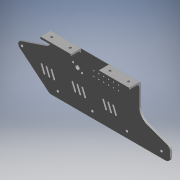
# Autodesk Inventor part: platform_track_support
Saved by Autodesk Inventor 2019 (Build 230136000, 136)
## iProperties
Part Number: platform_track_support
Material: Generic
Document SubType Name: Modeling
Designer: Jorge
Appearance: Default
Author: Jorge
Autodesk Inventor part; units mm, degrees
ref_plane "YZ Plane" through (0, 0, 0) normal (1, 0, 0) x (0, 1, 0)
ref_plane "XZ Plane" through (0, 0, 0) normal (0, 1, 0) x (-1, 0, 0)
ref_plane "XY Plane" through (0, 0, 0) normal (0, 0, 1) x (1, 0, 0)
sketch "Sketch1" plane through (0, 0, 0) normal (0, 0, 1) x (1, 0, 0)
  line L0 (2.505, 0) -> (188, 0)
  line L1 (195, 7) -> (195, 17.0802)
  line L2 (190.371, 23.6664) -> (158.2256, 35.2388)
  line L3 (145, 54.0565) -> (145, 89)
  line L4 (145, 89) -> (1.5, 89)
  line L5 (1.5, 89) -> (1.5, 73.7111)
  line L6 (-5.3421, 64.2228) -> (-46.8948, 50.393)
  line L7 (-1.9362, 1.5893) -> (-48.8068, 40.0623)
  arc A0 (-46.8948, 50.393) -> (-48.8068, 40.0623) centre (-45, 44.7) ccw
  arc A1 (-1.9362, 1.5893) -> (2.505, 0) centre (2.505, 7) ccw
  arc A2 (188, 0) -> (195, 7) centre (188, 7) ccw
  arc A3 (195, 17.0802) -> (190.371, 23.6664) centre (188, 17.0802) ccw
  arc A4 (145, 54.0565) -> (158.2256, 35.2388) centre (165, 54.0565) ccw
  arc A5 (-5.3421, 64.2228) -> (1.5, 73.7111) centre (-8.5, 73.7111) ccw
  line L8 (13, 10) -> (181, 10) construction
  circle A6 centre (13, 10) radius 2
  circle A7 centre (181, 10) radius 2
  circle A8 centre (69, 10) radius 2
  circle A9 centre (125, 10) radius 2
  circle A10 centre (-45, 44.7) radius 2
  circle A11 centre (45, 59.2) radius 3.5
  circle A12 centre (52.2081, 55.1868) radius 1.75
  line L9 (52.2081, 55.1868) -> (48.058, 57.4974) construction
  circle A13 centre (37.7919, 63.2132) radius 1.75
  line L10 (41.942, 60.9026) -> (37.7919, 63.2132) construction
  line L11 (48.058, 57.4974) -> (41.942, 60.9026) construction
  arc A14 (-11.7614, 35.5207) -> (-14.5469, 34.4068) centre (-13.1542, 34.9637) ccw
  arc A15 (-9.2558, 25.2142) -> (-10.0917, 23.2645) centre (-8.6989, 23.8214) ccw construction
  line L12 (-13.1542, 34.9637) -> (-8.6989, 23.8214) construction
  line L13 (-14.5469, 34.4068) -> (-10.0917, 23.2645)
  line L14 (-7.3061, 24.3784) -> (-11.7614, 35.5207)
  arc A16 (-7.3061, 24.3784) -> (-9.2558, 25.2142) centre (-8.6989, 23.8214) ccw construction
  arc A17 (-10.0917, 23.2645) -> (-7.3061, 24.3784) centre (-8.6989, 23.8214) ccw
  arc A18 (-12.5973, 33.571) -> (-11.7614, 35.5207) centre (-13.1542, 34.9637) ccw construction
  arc A19 (-14.5469, 34.4068) -> (-12.5973, 33.571) centre (-13.1542, 34.9637) ccw construction
  line L15 (-10.9265, 29.3926) -> (151.0905, 29.3926) construction
  arc A20 (-4.5973, 33.571) -> (-3.7614, 35.5207) centre (-5.1542, 34.9637) ccw construction
  arc A21 (-6.5469, 34.4068) -> (-4.5973, 33.571) centre (-5.1542, 34.9637) ccw construction
  arc A22 (-3.7614, 35.5207) -> (-6.5469, 34.4068) centre (-5.1542, 34.9637) ccw
  arc A23 (0.6939, 24.3784) -> (-1.2558, 25.2142) centre (-0.6989, 23.8214) ccw construction
  arc A24 (-2.0917, 23.2645) -> (0.6939, 24.3784) centre (-0.6989, 23.8214) ccw
  arc A25 (-1.2558, 25.2142) -> (-2.0917, 23.2645) centre (-0.6989, 23.8214) ccw construction
  line L16 (0.6939, 24.3784) -> (-3.7614, 35.5207)
  line L17 (-6.5469, 34.4068) -> (-2.0917, 23.2645)
  arc A26 (3.4027, 33.571) -> (4.2386, 35.5207) centre (2.8458, 34.9637) ccw construction
  arc A27 (1.4531, 34.4068) -> (3.4027, 33.571) centre (2.8458, 34.9637) ccw construction
  arc A28 (4.2386, 35.5207) -> (1.4531, 34.4068) centre (2.8458, 34.9637) ccw
  arc A29 (8.6939, 24.3784) -> (6.7442, 25.2142) centre (7.3011, 23.8214) ccw construction
  arc A30 (5.9083, 23.2645) -> (8.6939, 24.3784) centre (7.3011, 23.8214) ccw
  arc A31 (6.7442, 25.2142) -> (5.9083, 23.2645) centre (7.3011, 23.8214) ccw construction
  line L18 (8.6939, 24.3784) -> (4.2386, 35.5207)
  line L19 (1.4531, 34.4068) -> (5.9083, 23.2645)
  arc A32 (54.2386, 35.5207) -> (51.4531, 34.4068) centre (52.8458, 34.9637) ccw
  arc A33 (53.4027, 33.571) -> (54.2386, 35.5207) centre (52.8458, 34.9637) ccw construction
  arc A34 (46.2386, 35.5207) -> (43.4531, 34.4068) centre (44.8458, 34.9637) ccw
  arc A35 (51.4531, 34.4068) -> (53.4027, 33.571) centre (52.8458, 34.9637) ccw construction
  line L20 (58.6939, 24.3784) -> (54.2386, 35.5207)
  line L21 (51.4531, 34.4068) -> (55.9083, 23.2645)
  line L22 (50.6939, 24.3784) -> (46.2386, 35.5207)
  line L23 (43.4531, 34.4068) -> (47.9083, 23.2645)
  arc A36 (45.4027, 33.571) -> (46.2386, 35.5207) centre (44.8458, 34.9637) ccw construction
  arc A37 (43.4531, 34.4068) -> (45.4027, 33.571) centre (44.8458, 34.9637) ccw construction
  arc A38 (38.2386, 35.5207) -> (35.4531, 34.4068) centre (36.8458, 34.9637) ccw
  line L24 (36.8458, 34.9637) -> (41.3011, 23.8214) construction
  line L25 (35.4531, 34.4068) -> (39.9083, 23.2645)
  line L26 (42.6939, 24.3784) -> (38.2386, 35.5207)
  arc A39 (37.4027, 33.571) -> (38.2386, 35.5207) centre (36.8458, 34.9637) ccw construction
  arc A40 (35.4531, 34.4068) -> (37.4027, 33.571) centre (36.8458, 34.9637) ccw construction
  arc A41 (58.6939, 24.3784) -> (56.7442, 25.2142) centre (57.3011, 23.8214) ccw construction
  arc A42 (55.9083, 23.2645) -> (58.6939, 24.3784) centre (57.3011, 23.8214) ccw
  arc A43 (56.7442, 25.2142) -> (55.9083, 23.2645) centre (57.3011, 23.8214) ccw construction
  arc A44 (48.7442, 25.2142) -> (47.9083, 23.2645) centre (49.3011, 23.8214) ccw construction
  arc A45 (42.6939, 24.3784) -> (40.7442, 25.2142) centre (41.3011, 23.8214) ccw construction
  arc A46 (40.7442, 25.2142) -> (39.9083, 23.2645) centre (41.3011, 23.8214) ccw construction
  arc A47 (50.6939, 24.3784) -> (48.7442, 25.2142) centre (49.3011, 23.8214) ccw construction
  arc A48 (47.9083, 23.2645) -> (50.6939, 24.3784) centre (49.3011, 23.8214) ccw
  arc A49 (39.9083, 23.2645) -> (42.6939, 24.3784) centre (41.3011, 23.8214) ccw
  arc A50 (104.2386, 35.5207) -> (101.4531, 34.4068) centre (102.8458, 34.9637) ccw
  arc A51 (103.4027, 33.571) -> (104.2386, 35.5207) centre (102.8458, 34.9637) ccw construction
  arc A52 (96.2386, 35.5207) -> (93.4531, 34.4068) centre (94.8458, 34.9637) ccw
  arc A53 (101.4531, 34.4068) -> (103.4027, 33.571) centre (102.8458, 34.9637) ccw construction
  line L27 (108.6939, 24.3784) -> (104.2386, 35.5207)
  line L28 (101.4531, 34.4068) -> (105.9083, 23.2645)
  line L29 (100.6939, 24.3784) -> (96.2386, 35.5207)
  line L30 (93.4531, 34.4068) -> (97.9083, 23.2645)
  arc A54 (95.4027, 33.571) -> (96.2386, 35.5207) centre (94.8458, 34.9637) ccw construction
  arc A55 (93.4531, 34.4068) -> (95.4027, 33.571) centre (94.8458, 34.9637) ccw construction
  arc A56 (88.2386, 35.5207) -> (85.4531, 34.4068) centre (86.8458, 34.9637) ccw
  line L31 (86.8458, 34.9637) -> (91.3011, 23.8214) construction
  line L32 (85.4531, 34.4068) -> (89.9083, 23.2645)
  line L33 (92.6939, 24.3784) -> (88.2386, 35.5207)
  arc A57 (87.4027, 33.571) -> (88.2386, 35.5207) centre (86.8458, 34.9637) ccw construction
  arc A58 (85.4531, 34.4068) -> (87.4027, 33.571) centre (86.8458, 34.9637) ccw construction
  arc A59 (108.6939, 24.3784) -> (106.7442, 25.2142) centre (107.3011, 23.8214) ccw construction
  arc A60 (105.9083, 23.2645) -> (108.6939, 24.3784) centre (107.3011, 23.8214) ccw
  arc A61 (106.7442, 25.2142) -> (105.9083, 23.2645) centre (107.3011, 23.8214) ccw construction
  arc A62 (98.7442, 25.2142) -> (97.9083, 23.2645) centre (99.3011, 23.8214) ccw construction
  arc A63 (92.6939, 24.3784) -> (90.7442, 25.2142) centre (91.3011, 23.8214) ccw construction
  arc A64 (90.7442, 25.2142) -> (89.9083, 23.2645) centre (91.3011, 23.8214) ccw construction
  arc A65 (100.6939, 24.3784) -> (98.7442, 25.2142) centre (99.3011, 23.8214) ccw construction
  arc A66 (97.9083, 23.2645) -> (100.6939, 24.3784) centre (99.3011, 23.8214) ccw
  arc A67 (89.9083, 23.2645) -> (92.6939, 24.3784) centre (91.3011, 23.8214) ccw
  circle A68 centre (111.4036, 67.8621) radius 1
  line L34 (111.4036, 67.8621) -> (111.4036, 49.7064) construction
  line L35 (111.4036, 67.8621) -> (82.8465, 67.8621) construction
  circle A69 centre (111.4036, 59.8621) radius 1
  circle A70 centre (103.4036, 67.8621) radius 1
  circle A71 centre (103.4036, 59.8621) radius 1
  circle A72 centre (95.4036, 67.8621) radius 1
  circle A73 centre (95.4036, 59.8621) radius 1
  circle A74 centre (87.4036, 67.8621) radius 1
  circle A75 centre (87.4036, 59.8621) radius 1
  circle A76 centre (79.4036, 67.8621) radius 1
  circle A77 centre (79.4036, 59.8621) radius 1
  circle A78 centre (71.4036, 67.8621) radius 1
  circle A79 centre (71.4036, 59.8621) radius 1
  circle A80 centre (45, 59.2) radius 12.5 construction
  point P0 (0, 0)
  point P1 (0, 0)
  point P2 (195, 0)
  point P3 (195, 22)
  point P4 (145, 40)
  point P5 (1.5, 66.5)
  point P6 (39.0735, 29.3926)
  point P7 (89.0735, 29.3926)
  dimension "d0" = 195
  dimension "d1" = 22
  dimension "d2" = 89
  dimension "d3" = 50
  dimension "d5" = 143.5
  dimension "d6" = 22.5
  dimension "d7" = 40
  dimension "d11" = 44.7
  dimension "d12" = 190
  dimension "d13" = 6
  dimension "d14" = 7
  dimension "d15" = 20
  dimension "d16" = 10
  dimension "d19" = 4
  dimension "d20" = 4
  dimension "d21" = 4
  dimension "d22" = 4
  dimension "d23" = 168
  dimension "d24" = 56
  dimension "d25" = 56
  dimension "d26" = 56
  dimension "d27" = 10
  dimension "d28" = 14
  dimension "d29" = 4
  dimension "d32" = 7
  dimension "d33" = 59.2
  dimension "d34" = 100
  dimension "d35" = 3.5
  dimension "d36" = 3.5
  dimension "d37" = 16.5
  dimension "d40" = 3
  dimension "d41" = 3
  dimension "d42" = 12
  dimension "d45" = 8
  dimension "d52" = 50
  dimension "d57" = 2
  dimension "d60" = 8
  dimension "d63" = 8
  dimension "d87" = 25
  constraints: 122 point on circle, 81 centre point, 72 end point, 19 point on line, 18 tangent, 7 horizontal, 6 coincident, 4 vertical, 2 collinear, 2 equal radius, 2 midpoint, 1 parallel, 1 perpendicular, 155 other
  measures "d0" distance of point (0, 0) point (195, 0)
  measures "d1" distance of point (195, 0) point (195, 22)
  measures "d2" distance between parallel lines of L0 L4
  measures "d3" distance between parallel lines of L1 L3
  measures "d5" distance between parallel lines of L3 L5
  measures "d6" distance of L4.end point (1.5, 66.5)
  measures "d7" distance from line of L0 point (145, 40)
  measures "d11" distance from line of L0 A0.centre
  measures "d12" distance from line of L3 A0.centre
  measures "d13" radius of A0
  measures "d14" radius of A1
  measures "d15" radius of A4
  measures "d16" radius of A5
  measures "d19" diameter of A6
  measures "d20" diameter of A7
  measures "d21" diameter of A8
  measures "d22" diameter of A9
  measures "d23" distance of L8.end A6.centre
  measures "d24" distance of L8.start A8.centre
  measures "d25" distance of L8.end A9.centre
  measures "d26" distance of A9.centre A8.centre
  measures "d27" distance between parallel lines of L0 L8
  measures "d28" distance from line of L1 L8.end
  measures "d29" diameter of A10
  measures "d32" diameter of A11
  measures "d33" distance from line of L0 A11.centre
  measures "d34" distance from line of L3 A11.centre
  measures "d35" diameter of A12
  measures "d36" diameter of A13
  measures "d37" distance of L10.end L9.start
  measures "d40" diameter of A14
  measures "d41" diameter of A15
  measures "d42" distance of L12.start L12.end
  measures "d45" distance of L14.end L16.end
  measures "d52" distance of A26.centre A32.centre
  measures "d57" diameter of A68
  measures "d60" distance of L34.start A69.centre
  measures "d63" distance of L34.start A70.centre
  measures "d87" diameter of A80
extrude "Extrusion4" add sketch "Sketch1" along normal blind 3
sketch "Sketch2" plane through (0, 0, 3) normal (0, 0, 1) x (1, 0, 0)
  line L0 (145, 89) -> (1.5, 89) construction
  line L1 (1.5, 89) -> (50.5, 89)
  line L2 (50.5, 89) -> (50.5, 86)
  line L3 (50.5, 86) -> (1.5, 86)
  line L4 (1.5, 86) -> (1.5, 89)
  line L5 (145, 89) -> (96, 89)
  line L6 (96, 89) -> (96, 86)
  line L7 (96, 86) -> (145, 86)
  line L8 (145, 86) -> (145, 89)
  point P0 (0, 0)
  dimension "d68" = 49
  dimension "d69" = 3
  dimension "d70" = 49
  dimension "d71" = 3
  constraints: 16 end point, 4 parallel, 2 horizontal, 2 perpendicular
  measures "d68" distance of L2.end L3.end
  measures "d69" distance of L1.end L2.end
  measures "d70" distance of L7.end L6.end
  measures "d71" distance of L6.end L5.end
extrude "Extrusion5" add sketch "Sketch2" along normal blind 16.5
sketch "Sketch3" plane through (1.5, 89, 0) normal (0, 1, 0) x (1, 0, 0)
  circle A0 centre (134, -11.25) radius 2
  circle A1 centre (104, -11.25) radius 2
  line L0 (143.5, 0) -> (143.5, -19.5) construction
  line L1 (143.5, -11.25) -> (0, -11.25) construction
  line L2 (0, 0) -> (0, -19.5) construction
  line L3 (143.5, -3) -> (94.5, -3) construction
  line L4 (143.5, -19.5) -> (94.5, -19.5) construction
  circle A2 centre (39.5, -11.25) radius 2
  circle A3 centre (9.5, -11.25) radius 2
  line L5 (94.5, -19.5) -> (143.5, -19.5) construction
  line L6 (119, -19.5) -> (119, -3) construction
  line L7 (1.005, -3) -> (186.5, -3) construction
  line L8 (49, -19.5) -> (0, -19.5) construction
  line L9 (24.5, -19.5) -> (24.5, -3) construction
  point P0 (-1.5, 0)
  dimension "d74" = 4
  dimension "d75" = 4
  dimension "d76" = 16.5
  dimension "d77" = 8.25
  dimension "d78" = 4
  dimension "d79" = 4
  dimension "d80" = 30
  dimension "d81" = 30
  constraints: 8 point on line, 6 end point, 4 centre point, 2 midpoint, 2 perpendicular, 2 symmetric about line, 1 horizontal
  measures "d74" diameter of A0
  measures "d75" diameter of A1
  measures "d76" distance between parallel lines of L4 L3
  measures "d77" distance between parallel lines of L4 L1
  measures "d78" diameter of A2
  measures "d79" diameter of A3
  measures "d80" distance of A1.centre A0.centre
  measures "d81" distance of A2.centre A3.centre
extrude "Extrusion6" cut sketch "Sketch3" against normal through all
fillet "Fillet1" radius 4.5 1 edges at (73.25, 89, 0)
fillet "Fillet2" radius 4.5 1 edges at (26, 86, 3)
fillet "Fillet3" radius 4.5 1 edges at (120.5, 86, 3)
body "Solid4"
